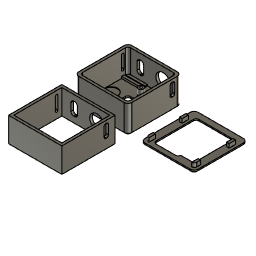
Action_2_Poor_3DP (Autodesk Fusion 360 design; units mm, degrees)
Autodesk Fusion 360 part; units mm, degrees
box "长方体基本要素1" add length 41 width 41 height 2 placed x (0, 1, 0) y (-1, 0, 0) z (0, 0, 1) at (41, 0, 0) makes body 1
sketch "草图2" plane through (0, 0, 0) normal (0, 0, 1) x (1, 0, 0)
  line L0 (0, 41) -> (41, 41)
  line L1 (41, 41) -> (41, 0)
  line L2 (41, 0) -> (0, 0)
  line L3 (0, 0) -> (0, 41)
  line L4 (4.5, 6.5, 2) -> (2, 6.5, 2)
  line L5 (2, 6.5, 2) -> (2, 2, 2)
  line L6 (2, 2, 2) -> (6.5, 2, 2)
  line L7 (6.5, 2, 2) -> (6.5, 4.5, 2)
  line L8 (39, 2, 2) -> (34.5, 2, 2)
  line L9 (34.5, 2, 2) -> (34.5, 4.5, 2)
  line L10 (36.5, 6.5, 2) -> (39, 6.5, 2)
  line L11 (39, 6.5, 2) -> (39, 2, 2)
  circle A0 through (22.5, 30.5, 2) (19.5, 32.2321, 2) (19.5, 28.7679, 2)
  arc A1 through (36.5, 6.5, 2) (35.0858, 5.9142, 2) (34.5, 4.5, 2)
  arc A2 through (6.5, 4.5, 2) (5.9142, 5.9142, 2) (4.5, 6.5, 2)
  line L12 (-10, 25) -> (-10, 25)
  line L13 (12, 21, 2) -> (12, 16, 2)
  line L14 (-10, 10) -> (-10, 10)
  line L15 (2, 16, 2) -> (2, 21, 2)
  arc A3 through (7, 26, 2) (3.4645, 24.5355, 2) (2, 21, 2)
  arc A4 through (12, 21, 2) (10.5355, 24.5355, 2) (7, 26, 2)
  arc A5 through (7, 11, 2) (10.5355, 12.4645, 2) (12, 16, 2)
  arc A6 through (2, 16, 2) (3.4645, 12.4645, 2) (7, 11, 2)
  circle A7 centre (4.5, 14.5) radius 0.75
  circle A8 centre (36.5, 9.5) radius 0.75
  line L16 (17.5, 25.5, 2) -> (23.5, 25.5, 2)
  line L17 (25.5, 23.5, 2) -> (25.5, 17.5, 2)
  line L18 (23.5, 15.5, 2) -> (17.5, 15.5, 2)
  line L19 (15.5, 17.5, 2) -> (15.5, 23.5, 2)
  arc A9 through (17.5, 25.5, 2) (16.0858, 24.9142, 2) (15.5, 23.5, 2)
  arc A10 through (25.5, 23.5, 2) (24.9142, 24.9142, 2) (23.5, 25.5, 2)
  arc A11 through (23.5, 15.5, 2) (24.9142, 16.0858, 2) (25.5, 17.5, 2)
  arc A12 through (15.5, 17.5, 2) (16.0858, 16.0858, 2) (17.5, 15.5, 2)
  circle A13 centre (20.5, 20.5) radius 14.8
  dimension "d42" = 2
  dimension "d43" = 2
  dimension "d95" = 5
  dimension "d106" = 1.5
  dimension "d107" = 1.5
  dimension "d140" = 2
  constraint horizontal L0
  constraint vertical L1
  constraint horizontal L2
  constraint vertical L3
  measures "d106" diameter of A7
  measures "d107" diameter of A8
extrude "拉伸22" cut sketch "草图2" along normal blind 0.8 contours A13 bodies 1
extrude "拉伸17" cut sketch "草图2" against normal blind 2 contours L16 L17 L18 L19 A9 A10 A11 A12 in plane through (0, 0, 2) normal (0, 0, 1) bodies 1
extrude "拉伸14" cut sketch "草图2" along normal blind 2 contours A8 bodies 1
extrude "拉伸15" cut sketch "草图2" along normal blind 2 contours A7 bodies 1
box "长方体基本要素9" add length 2 width 15 height 1 placed x (0, -1, 0) y (1, 0, 0) z (0, 0, 1) at (2, 39, 2) bodies 1
box "长方体基本要素10" add length 2 width 15 height 1.5 placed x (0, -1, 0) y (1, 0, 0) z (0, 0, 1) at (2, 36, 2) bodies 1
box "长方体基本要素11" add length 2 width 5 height 1 placed x (0, -1, 0) y (1, 0, 0) z (0, 0, 1) at (34, 39, 2) bodies 1
box "长方体基本要素12" add length 2 width 5 height 1.5 placed x (0, -1, 0) y (1, 0, 0) z (0, 0, 1) at (34, 36, 2) bodies 1
extrude "拉伸27" cut sketch "草图2" against normal blind 0.4 contours L13 L15 A3 A4 A5 A6 in plane through (0, 0, 2) normal (0, 0, 1) bodies 1
extrude "拉伸28" add sketch "草图2" along normal blind 5 contours L4 L5 L6 L7 A2 | L8 L9 L10 L11 A1 | A0 in plane through (0, 0, 2) normal (0, 0, 1) bodies 1
hole "孔8" at (20.5, 30.5, 7) direction (0, 0, -1) diameter 1.623 depth 4 tip angle 180 bodies 1
thread "螺纹8" "ISO Metric profile 2.0 M2x0.4 6H" major diameter 2.074 minor diameter 1.623 pitch 0.4 angle 60 resizes the face on face at (20.5405, 31.3105, 5.6667) on bodies 1
hole "孔9" at (4.5, 4.5, 7) direction (0, 0, -1) diameter 1.623 depth 4 tip angle 180 bodies 1
thread "螺纹9" "ISO Metric profile 2.0 M2x0.4 6H" major diameter 2.074 minor diameter 1.623 pitch 0.4 angle 60 resizes the face on face at (4.5808, 3.6925, 4.3333) on bodies 1
hole "孔10" at (36.5, 4.5, 7) direction (0, 0, -1) diameter 1.623 depth 4 tip angle 180 bodies 1
thread "螺纹10" "ISO Metric profile 2.0 M2x0.4 6H" major diameter 2.074 minor diameter 1.623 pitch 0.4 angle 60 resizes the face on face at (36.0769, 3.8076, 5.6667) on bodies 1
box "长方体基本要素2" add length 41 width 41 height 19 placed x (0, -1, 0) y (1, 0, 0) z (0, 0, 1) at (0, -10, 0) separate body makes body 2
shell "抽壳1" thickness 2 removed faces 2 at (27.3333, -23.6667, 19) at (27.3333, -23.6667, 0) on bodies 2
sketch "草图7" plane through (41, 0, 0) normal (1, 0, 0) x (0, 1, 0)
  line L0 (-51, 19) -> (-51, 0)
  line L1 (-51, 0) -> (-10, 0)
  line L2 (-10, 0) -> (-10, 19)
  line L3 (-10, 19) -> (-51, 19)
  circle A0 centre (-46.4, 16.5) radius 1
  circle A1 centre (-21, 16.5) radius 1
  line L4 (-17, 17) -> (-16.5, 17)
  line L5 (-15, 15.5) -> (-15, 8.5)
  line L6 (-16.5, 7) -> (-17, 7)
  line L7 (-18.5, 8.5) -> (-18.5, 15.5)
  arc A2 (-17, 17) -> (-18.5, 15.5) centre (-17, 15.5) ccw
  arc A3 (-15, 15.5) -> (-16.5, 17) centre (-16.5, 15.5) ccw
  arc A4 (-16.5, 7) -> (-15, 8.5) centre (-16.5, 8.5) ccw
  arc A5 (-18.5, 8.5) -> (-17, 7) centre (-17, 8.5) ccw
  dimension "d195" = 1.5
  constraint horizontal L4
  constraint vertical L5
  constraint horizontal L6
  constraint vertical L7
  constraint tangent L4 A2
  constraint tangent L7 A2
  constraint tangent L4 A3
  constraint tangent L5 A3
  constraint equal A2 A3
  constraint tangent L5 A4
  constraint tangent L6 A4
  constraint equal A2 A4
  constraint tangent L6 A5
  constraint tangent L7 A5
  constraint equal A2 A5
  measures "d195" radius of A2
sketch "草图8" plane through (0, 0, 0) normal (-1, 0, 0) x (0, -1, 0)
  line L0 (10, 19) -> (10, 0)
  line L1 (10, 0) -> (51, 0)
  line L2 (51, 0) -> (51, 19)
  line L3 (51, 19) -> (10, 19)
  circle A0 centre (46.4, 16.5) radius 1
  circle A1 centre (19.5, 16.5) radius 1
  line L4 (16, 5) -> (16, 5)
  line L5 (15, 5.5) -> (15, 15.5)
  line L6 (16, 17) -> (16, 17)
  line L7 (17, 15.5) -> (17, 5.5)
  arc A2 (16, 16.5) -> (15, 15.5) centre (16, 15.5) ccw
  arc A3 (17, 15.5) -> (16, 16.5) centre (16, 15.5) ccw
  arc A4 (16, 4.5) -> (17, 5.5) centre (16, 5.5) ccw
  arc A5 (15, 5.5) -> (16, 4.5) centre (16, 5.5) ccw
  dimension "d157" = 1
  constraint vertical L5
  constraint vertical L7
  constraint tangent L5 A2
  constraint tangent L7 A3
  constraint equal A2 A3
  constraint tangent L7 A4
  constraint equal A2 A4
  constraint tangent L5 A5
  constraint equal A2 A5
  measures "d157" radius of A2
sketch "草图17" plane through (0, -10, 0) normal (0, 1, 0) x (-1, 0, 0)
  line L0 (-41, 19) -> (-41, 0)
  line L1 (-41, 0) -> (0, 0)
  line L2 (0, 0) -> (0, 19)
  line L3 (0, 19) -> (-41, 19)
  circle A0 centre (-29, 9.5) radius 5.5
  line L4 (-12, 14.5) -> (-11, 14.5)
  line L5 (-9, 12.5) -> (-9, 6.5)
  line L6 (-11, 4.5) -> (-12, 4.5)
  line L7 (-14, 6.5) -> (-14, 12.5)
  arc A1 (-12, 14.5) -> (-14, 12.5) centre (-12, 12.5) ccw
  arc A2 (-9, 12.5) -> (-11, 14.5) centre (-11, 12.5) ccw
  arc A3 (-11, 4.5) -> (-9, 6.5) centre (-11, 6.5) ccw
  arc A4 (-14, 6.5) -> (-12, 4.5) centre (-12, 6.5) ccw
  dimension "d144" = 2
  constraint horizontal L4
  constraint vertical L5
  constraint horizontal L6
  constraint vertical L7
  constraint tangent L4 A1
  constraint tangent L7 A1
  constraint tangent L4 A2
  constraint tangent L5 A2
  constraint equal A1 A2
  constraint tangent L5 A3
  constraint tangent L6 A3
  constraint equal A1 A3
  constraint tangent L6 A4
  constraint tangent L7 A4
  constraint equal A1 A4
  measures "d144" radius of A1
extrude "拉伸30" cut sketch "草图7" against normal blind 2 contours L4 L5 L6 L7 A2 A3 A4 A5 bodies 2
extrude "拉伸21" cut sketch "草图8" against normal blind 2 contours L5 L7 A2 A3 A4 A5 bodies 2
extrude "拉伸18" cut sketch "草图17" against normal blind 2 contours A0 | L4 L5 L6 L7 A1 A2 A3 A4 bodies 2
boxprimitive "长方体基本要素8" [suppressed]
sketch "草图4" plane through (0, 0, 0) normal (0, 0, 1) x (1, 0, 0)
  line L0 (51, 0) -> (92, 0)
  line L1 (92, 0) -> (92, 41)
  line L2 (92, 41) -> (51, 41)
  line L3 (51, 41) -> (51, 0)
  line L4 (89.9, 2.1, 2) -> (87.9, 2.1, 2)
  line L5 (87.9, 2.1, 2) -> (87.9, 7.1, 2)
  line L6 (87.9, 7.1, 2) -> (89.9, 7.1, 2)
  line L7 (89.9, 7.1, 2) -> (89.9, 2.1, 2)
  line L8 (55.1, 2.1, 2) -> (53.1, 2.1, 2)
  line L9 (53.1, 2.1, 2) -> (53.1, 7.1, 2)
  line L10 (53.1, 7.1, 2) -> (55.1, 7.1, 2)
  line L11 (55.1, 7.1, 2) -> (55.1, 2.1, 2)
  line L12 (87.9, 34, 2) -> (89.9, 34, 2)
  line L13 (89.9, 34, 2) -> (89.9, 29, 2)
  line L14 (89.9, 29, 2) -> (87.9, 29, 2)
  line L15 (87.9, 29, 2) -> (87.9, 34, 2)
  line L16 (55.1, 32.5, 2) -> (53.1, 32.5, 2)
  line L17 (53.1, 32.5, 2) -> (53.1, 27.5, 2)
  line L18 (53.1, 27.5, 2) -> (55.1, 27.5, 2)
  line L19 (55.1, 27.5, 2) -> (55.1, 32.5, 2)
  line L20 (56.5, 39) -> (86.5, 39)
  line L21 (88.5, 37) -> (88.5, 5.6)
  line L22 (86.5, 3.6) -> (56.5, 3.6)
  line L23 (54.5, 5.6) -> (54.5, 37)
  line L24 (59, 36.5, 2) -> (84, 36.5, 2)
  line L25 (86, 34.5, 2) -> (86, 7.6, 2)
  line L26 (84, 5.6, 2) -> (76, 5.6, 2)
  line L27 (57, 5.6, 2) -> (57, 34.5, 2)
  line L28 (76, 5.6, 2) -> (76, 5.6, 2)
  line L29 (74, 3.6, 2) -> (59, 3.6, 2)
  line L30 (57, 5.6, 2) -> (57, 5.6, 2)
  arc A0 (56.5, 39) -> (54.5, 37) centre (56.5, 37) ccw
  arc A1 (88.5, 37) -> (86.5, 39) centre (86.5, 37) ccw
  arc A2 (86.5, 3.6) -> (88.5, 5.6) centre (86.5, 5.6) ccw
  arc A3 (54.5, 5.6) -> (56.5, 3.6) centre (56.5, 5.6) ccw
  arc A4 through (59, 36.5, 2) (57.5858, 35.9142, 2) (57, 34.5, 2)
  arc A5 through (86, 34.5, 2) (85.4142, 35.9142, 2) (84, 36.5, 2)
  arc A6 through (84, 5.6, 2) (85.4142, 6.1858, 2) (86, 7.6, 2)
  arc A7 through (57, 5.6, 2) (57.5858, 4.1858, 2) (59, 3.6, 2)
  arc A8 through (74, 3.6, 2) (75.4142, 4.1858, 2) (76, 5.6, 2)
  point P0 (54.5, 39)
  point P1 (88.5, 3.6)
  point P2 (57, 36.5)
  point P3 (86, 5.6)
  dimension "d164" = 2
  constraint horizontal L0
  constraint vertical L1
  constraint horizontal L2
  constraint vertical L3
  constraint horizontal L20
  constraint vertical L21
  constraint horizontal L22
  constraint vertical L23
  constraint tangent L20 A0
  constraint tangent L23 A0
  constraint tangent L20 A1
  constraint tangent L21 A1
  constraint equal A0 A1
  constraint tangent L21 A2
  constraint tangent L22 A2
  constraint equal A0 A2
  constraint tangent L22 A3
  constraint tangent L23 A3
  constraint equal A0 A3
  measures "d164" radius of A0
box "长方体基本要素3" add length 41 width 41 height 2 placed x (0, 1, 0) y (-1, 0, 0) z (0, 0, 1) at (92, 0, 0) separate body makes body 3
extrude "拉伸23" cut sketch "草图4" against normal blind 2 contours L24 L25 L26 L27 L29 A4 A5 A6 A7 A8 in plane through (0, 0, 2) normal (0, 0, 1) bodies 3
extrude "拉伸24" cut sketch "草图4" along normal blind 1 contours L20 L21 L22 L23 A0 A1 A2 A3 bodies 3
extrude "拉伸29" add sketch "草图4" along normal blind 3 contours L4 L5 L6 L7 | L8 L9 L10 L11 | L12 L13 L14 L15 | L16 L17 L18 L19 in plane through (0, 0, 2) normal (0, 0, 1) bodies 3
copy_body "复制和粘贴实体3" bodies 2 makes body 4
move_body "移动8" bodies 4 to x (1, 0, 0) y (0, 1, 0) z (0, 0, 1) at (0, 51, 2)
combine "合并1" operation add target body 1 tool bodies 4
fillet "圆角4" radius 3 8 edges at (41, 0, 10.5) (41, 41, 10.5) (0, 0, 10.5) (0, 41, 10.5) (51, 0, 1) (92, 0, 1) (92, 41, 1) (51, 41, 1) on bodies 1 3
fillet "圆角6" radius 2 6 edges at (2, 39, 12) (2, 2, 14) (39, 2, 14) (39, 39, 12) (53.1, 2.1, 3.5) (89.9, 2.1, 3.5) on bodies 1 3
chamfer "倒角3" distance 1 angle 45 16 edges at (20.5, 0, 0) (0.8787, 0.8787, 0) (0, 20.5, 0) (0.8787, 40.1213, 0) (20.5, 41, 0) (40.1213, 40.1213, 0) (41, 20.5, 0) (40.1213, 0.8787, 0) (71.5, 0, 0) (51.8787, 0.8787, 0) (51, 20.5, 0) (51.8787, 40.1213, 0) (71.5, 41, 0) (91.1213, 40.1213, 0) (92, 20.5, 0) (91.1213, 0.8787, 0) on bodies 1 3
named bodies: "前壳", "侧壳", "后壳", "侧壳 (1)"
